Autodesk Fusion 360 part; units mm, degrees
(part 4 of 8)
  spline S174 degree 5 poles (79.544, 19.9185) (79.5234, 19.9219) (79.4821, 19.9288) (79.4202, 19.939) (79.3377, 19.9523) (79.2346, 19.9687) (79.1314, 19.9847) (79.0284, 20.0004) (78.9253, 20.0157) (78.8222, 20.0307) (78.7192, 20.0453) (78.6162, 20.0596) (78.5133, 20.0735) (78.4103, 20.087) (78.3074, 20.1002) (78.2045, 20.113) (78.1017, 20.1254) (77.9989, 20.1375) (77.8961, 20.1491) (77.7934, 20.1604) (77.6906, 20.1714) (77.588, 20.1819) (77.4853, 20.192) (77.3827, 20.2018) (77.2802, 20.2111) (77.1777, 20.2201) (77.0752, 20.2287) (76.9728, 20.2368) (76.8704, 20.2446) (76.768, 20.2519) (76.6658, 20.2588) (76.5635, 20.2653) (76.4613, 20.2714) (76.3592, 20.277) (76.2571, 20.2822) (76.1551, 20.287) (76.0531, 20.2913) (75.9512, 20.2952) (75.8646, 20.2981) (75.7985, 20.3001) (75.7526, 20.3014) (75.7272, 20.302) (75.722, 20.3022) knots -1 -1 -1 -1 -1 -1 -0.985714 -0.971429 -0.957143 -0.942857 -0.928571 -0.914286 -0.9 -0.885714 -0.871429 -0.857143 -0.842857 -0.828571 -0.814286 -0.8 -0.785714 -0.771429 -0.757143 -0.742857 -0.728571 -0.714286 -0.7 -0.685714 -0.671429 -0.657143 -0.642857 -0.628571 -0.614286 -0.6 -0.585714 -0.571429 -0.557143 -0.542857 -0.528571 -0.514286 -0.5 -0.485714 -0.471429 -0.467834 -0.467834 -0.467834 -0.467834 -0.467834 -0.467834
  spline S175 degree 3 poles (74.7851, 21.0311) (74.8203, 20.9058) (74.8797, 20.7885) (75.0401, 20.5833) (75.1396, 20.4974) (75.3241, 20.3923) (75.4002, 20.3606) (75.5584, 20.3165) (75.6399, 20.3043) (75.722, 20.3022) knots 0 0 0 0 0.039064 0.039064 0.078129 0.078129 0.102767 0.102767 0.127404 0.127404 0.127404 0.127404
  arc A88 (74.7851, 21.0311) -> (74.7535, 21.1431) centre (0, 0) ccw
  spline S176 degree 3 poles (75.1715, 22.2542) (75.0623, 22.1834) (74.9679, 22.0918) (74.8196, 21.8778) (74.767, 21.7573) (74.7214, 21.5499) (74.7137, 21.4678) (74.7186, 21.3036) (74.7311, 21.2221) (74.7535, 21.1431) knots 0 0 0 0 0.039064 0.039064 0.078129 0.078129 0.102767 0.102767 0.127404 0.127404 0.127404 0.127404
  spline S177 degree 5 poles (75.1715, 22.2542) (75.1758, 22.257) (75.1972, 22.2709) (75.2356, 22.2959) (75.291, 22.3322) (75.3633, 22.3799) (75.4482, 22.4364) (75.5328, 22.4934) (75.6173, 22.5508) (75.7016, 22.6086) (75.7858, 22.6667) (75.8697, 22.7253) (75.9535, 22.7843) (76.0371, 22.8436) (76.1205, 22.9033) (76.2038, 22.9634) (76.2868, 23.0239) (76.3697, 23.0847) (76.4525, 23.1459) (76.535, 23.2075) (76.6174, 23.2694) (76.6996, 23.3317) (76.7817, 23.3943) (76.8635, 23.4573) (76.9452, 23.5206) (77.0268, 23.5843) (77.1081, 23.6483) (77.1893, 23.7126) (77.2704, 23.7773) (77.3512, 23.8423) (77.4319, 23.9076) (77.5125, 23.9733) (77.5928, 24.0392) (77.673, 24.1055) (77.7531, 24.1721) (77.8329, 24.239) (77.9127, 24.3063) (77.9922, 24.3738) (78.0716, 24.4417) (78.135, 24.4962) (78.1824, 24.5372) (78.214, 24.5646) (78.2298, 24.5784) knots 0.467834 0.467834 0.467834 0.467834 0.467834 0.467834 0.471429 0.485714 0.5 0.514286 0.528571 0.542857 0.557143 0.571429 0.585714 0.6 0.614286 0.628571 0.642857 0.657143 0.671429 0.685714 0.7 0.714286 0.728571 0.742857 0.757143 0.771429 0.785714 0.8 0.814286 0.828571 0.842857 0.857143 0.871429 0.885714 0.9 0.914286 0.928571 0.942857 0.957143 0.971429 0.985714 1 1 1 1 1 1
  arc A89 (78.2298, 24.5784) -> (77.736, 26.098) centre (0, 0) ccw
  spline S178 degree 5 poles (77.736, 26.098) (77.7152, 26.0998) (77.6735, 26.1034) (77.611, 26.1087) (77.5277, 26.1156) (77.4236, 26.1238) (77.3195, 26.1317) (77.2155, 26.1393) (77.1116, 26.1464) (77.0077, 26.1533) (76.9038, 26.1598) (76.8, 26.1659) (76.6963, 26.1717) (76.5926, 26.1771) (76.489, 26.1821) (76.3854, 26.1868) (76.2819, 26.1912) (76.1785, 26.1951) (76.0751, 26.1987) (75.9718, 26.2019) (75.8685, 26.2047) (75.7653, 26.2072) (75.6622, 26.2092) (75.5592, 26.2109) (75.4562, 26.2122) (75.3533, 26.2131) (75.2505, 26.2136) (75.1477, 26.2136) (75.045, 26.2133) (74.9424, 26.2126) (74.8399, 26.2115) (74.7375, 26.2099) (74.6352, 26.208) (74.5329, 26.2056) (74.4307, 26.2028) (74.3286, 26.1995) (74.2267, 26.1959) (74.1248, 26.1917) (74.0382, 26.1878) (73.9721, 26.1846) (73.9263, 26.1823) (73.9008, 26.1809) (73.8957, 26.1807) knots -1 -1 -1 -1 -1 -1 -0.985714 -0.971429 -0.957143 -0.942857 -0.928571 -0.914286 -0.9 -0.885714 -0.871429 -0.857143 -0.842857 -0.828571 -0.814286 -0.8 -0.785714 -0.771429 -0.757143 -0.742857 -0.728571 -0.714286 -0.7 -0.685714 -0.671429 -0.657143 -0.642857 -0.628571 -0.614286 -0.6 -0.585714 -0.571429 -0.557143 -0.542857 -0.528571 -0.514286 -0.5 -0.485714 -0.471429 -0.467834 -0.467834 -0.467834 -0.467834 -0.467834 -0.467834
  spline S179 degree 3 poles (72.9045, 26.8339) (72.9494, 26.7117) (73.0178, 26.5994) (73.1939, 26.4075) (73.2998, 26.3296) (73.4919, 26.2393) (73.5703, 26.2136) (73.7315, 26.1821) (73.8137, 26.1763) (73.8957, 26.1807) knots 0 0 0 0 0.039064 0.039064 0.078129 0.078129 0.102767 0.102767 0.127404 0.127404 0.127404 0.127404
  arc A90 (72.9045, 26.8339) -> (72.8642, 26.943) centre (0, 0) ccw
  spline S180 degree 3 poles (73.1937, 28.0835) (73.0904, 28.0043) (73.0035, 27.9056) (72.8724, 27.6806) (72.8295, 27.5563) (72.8003, 27.346) (72.7991, 27.2636) (72.8168, 27.1003) (72.8357, 27.0201) (72.8642, 26.943) knots 0 0 0 0 0.039064 0.039064 0.078129 0.078129 0.102767 0.102767 0.127404 0.127404 0.127404 0.127404
  spline S181 degree 5 poles (73.1937, 28.0835) (73.1978, 28.0866) (73.218, 28.1021) (73.2543, 28.1301) (73.3067, 28.1706) (73.3751, 28.2238) (73.4552, 28.2869) (73.5352, 28.3503) (73.6149, 28.4141) (73.6944, 28.4784) (73.7737, 28.543) (73.8528, 28.6079) (73.9317, 28.6733) (74.0104, 28.739) (74.0889, 28.8051) (74.1672, 28.8715) (74.2452, 28.9383) (74.3231, 29.0055) (74.4008, 29.073) (74.4783, 29.1408) (74.5555, 29.209) (74.6326, 29.2776) (74.7095, 29.3464) (74.7861, 29.4156) (74.8626, 29.4852) (74.9389, 29.555) (75.015, 29.6252) (75.0909, 29.6957) (75.1666, 29.7666) (75.2421, 29.8377) (75.3175, 29.9091) (75.3926, 29.9809) (75.4675, 30.053) (75.5423, 30.1254) (75.6169, 30.198) (75.6912, 30.271) (75.7654, 30.3443) (75.8394, 30.4179) (75.9132, 30.4917) (75.9721, 30.5511) (76.0162, 30.5957) (76.0456, 30.6255) (76.0603, 30.6404) knots 0.467834 0.467834 0.467834 0.467834 0.467834 0.467834 0.471429 0.485714 0.5 0.514286 0.528571 0.542857 0.557143 0.571429 0.585714 0.6 0.614286 0.628571 0.642857 0.657143 0.671429 0.685714 0.7 0.714286 0.728571 0.742857 0.757143 0.771429 0.785714 0.8 0.814286 0.828571 0.842857 0.857143 0.871429 0.885714 0.9 0.914286 0.928571 0.942857 0.957143 0.971429 0.985714 1 1 1 1 1 1
  arc A91 (76.0603, 30.6404) -> (75.4488, 32.1167) centre (0, 0) ccw
  spline S182 degree 5 poles (75.4488, 32.1167) (75.4279, 32.1168) (75.386, 32.1172) (75.3233, 32.1175) (75.2397, 32.1178) (75.1353, 32.1179) (75.0309, 32.1176) (74.9266, 32.1169) (74.8224, 32.116) (74.7183, 32.1146) (74.6143, 32.1129) (74.5103, 32.1109) (74.4065, 32.1085) (74.3027, 32.1058) (74.199, 32.1027) (74.0953, 32.0992) (73.9918, 32.0954) (73.8884, 32.0912) (73.785, 32.0867) (73.6818, 32.0818) (73.5786, 32.0765) (73.4756, 32.0708) (73.3726, 32.0648) (73.2698, 32.0584) (73.167, 32.0516) (73.0644, 32.0444) (72.9618, 32.0368) (72.8594, 32.0289) (72.757, 32.0205) (72.6548, 32.0117) (72.5527, 32.0026) (72.4507, 31.993) (72.3488, 31.983) (72.2471, 31.9726) (72.1454, 31.9618) (72.0439, 31.9505) (71.9425, 31.9389) (71.8413, 31.9267) (71.7553, 31.9161) (71.6896, 31.9077) (71.6442, 31.9018) (71.6189, 31.8984) (71.6138, 31.8977) knots -1 -1 -1 -1 -1 -1 -0.985714 -0.971429 -0.957143 -0.942857 -0.928571 -0.914286 -0.9 -0.885714 -0.871429 -0.857143 -0.842857 -0.828571 -0.814286 -0.8 -0.785714 -0.771429 -0.757143 -0.742857 -0.728571 -0.714286 -0.7 -0.685714 -0.671429 -0.657143 -0.642857 -0.628571 -0.614286 -0.6 -0.585714 -0.571429 -0.557143 -0.542857 -0.528571 -0.514286 -0.5 -0.485714 -0.471429 -0.467834 -0.467834 -0.467834 -0.467834 -0.467834 -0.467834
  spline S183 degree 3 poles (70.5744, 32.4711) (70.6288, 32.3529) (70.7058, 32.2463) (70.8963, 32.0688) (71.008, 31.9995) (71.2067, 31.9245) (71.2868, 31.9051) (71.45, 31.8863) (71.5324, 31.887) (71.6138, 31.8977) knots 0 0 0 0 0.039064 0.039064 0.078129 0.078129 0.102767 0.102767 0.127404 0.127404 0.127404 0.127404
  arc A92 (70.5744, 32.4711) -> (70.5256, 32.5768) centre (0, 0) ccw
  spline S184 degree 3 poles (70.7647, 33.7396) (70.6679, 33.6526) (70.589, 33.5474) (70.476, 33.3128) (70.443, 33.1855) (70.4303, 32.9736) (70.4356, 32.8913) (70.4661, 32.7299) (70.4912, 32.6514) (70.5256, 32.5768) knots 0 0 0 0 0.039064 0.039064 0.078129 0.078129 0.102767 0.102767 0.127404 0.127404 0.127404 0.127404
  spline S185 degree 5 poles (70.7647, 33.7396) (70.7685, 33.7431) (70.7874, 33.7601) (70.8215, 33.7908) (70.8705, 33.8353) (70.9345, 33.8938) (71.0094, 33.9629) (71.0842, 34.0324) (71.1586, 34.1023) (71.2329, 34.1726) (71.3069, 34.2432) (71.3806, 34.3142) (71.4541, 34.3855) (71.5274, 34.4572) (71.6005, 34.5292) (71.6733, 34.6016) (71.7459, 34.6743) (71.8183, 34.7474) (71.8904, 34.8208) (71.9623, 34.8945) (72.034, 34.9686) (72.1054, 35.0429) (72.1767, 35.1176) (72.2477, 35.1926) (72.3185, 35.2679) (72.389, 35.3436) (72.4594, 35.4195) (72.5295, 35.4958) (72.5995, 35.5723) (72.6692, 35.6491) (72.7386, 35.7263) (72.8079, 35.8037) (72.877, 35.8815) (72.9458, 35.9595) (73.0144, 36.0378) (73.0829, 36.1164) (73.1511, 36.1952) (73.2191, 36.2744) (73.2869, 36.3538) (73.3409, 36.4176) (73.3814, 36.4656) (73.4083, 36.4976) (73.4218, 36.5136) knots 0.467834 0.467834 0.467834 0.467834 0.467834 0.467834 0.471429 0.485714 0.5 0.514286 0.528571 0.542857 0.557143 0.571429 0.585714 0.6 0.614286 0.628571 0.642857 0.657143 0.671429 0.685714 0.7 0.714286 0.728571 0.742857 0.757143 0.771429 0.785714 0.8 0.814286 0.828571 0.842857 0.857143 0.871429 0.885714 0.9 0.914286 0.928571 0.942857 0.957143 0.971429 0.985714 1 1 1 1 1 1
  arc A93 (73.4218, 36.5136) -> (72.6964, 37.9373) centre (0, 0) ccw
  spline S186 degree 5 poles (72.6964, 37.9373) (72.6755, 37.9358) (72.6338, 37.9329) (72.5712, 37.9283) (72.4878, 37.9221) (72.3837, 37.9139) (72.2797, 37.9054) (72.1758, 37.8966) (72.072, 37.8875) (71.9683, 37.878) (71.8647, 37.8681) (71.7612, 37.8579) (71.6579, 37.8474) (71.5546, 37.8365) (71.4515, 37.8253) (71.3485, 37.8137) (71.2456, 37.8018) (71.1428, 37.7895) (71.0401, 37.7769) (70.9376, 37.7639) (70.8351, 37.7505) (70.7328, 37.7368) (70.6307, 37.7227) (70.5286, 37.7082) (70.4267, 37.6934) (70.3249, 37.6782) (70.2233, 37.6626) (70.1218, 37.6466) (70.0204, 37.6302) (69.9192, 37.6135) (69.8182, 37.5963) (69.7172, 37.5788) (69.6164, 37.5608) (69.5158, 37.5425) (69.4153, 37.5237) (69.315, 37.5045) (69.2149, 37.4849) (69.1149, 37.4649) (69.03, 37.4475) (68.9652, 37.434) (68.9203, 37.4245) (68.8954, 37.4192) (68.8904, 37.4182) knots -1 -1 -1 -1 -1 -1 -0.985714 -0.971429 -0.957143 -0.942857 -0.928571 -0.914286 -0.9 -0.885714 -0.871429 -0.857143 -0.842857 -0.828571 -0.814286 -0.8 -0.785714 -0.771429 -0.757143 -0.742857 -0.728571 -0.714286 -0.7 -0.685714 -0.671429 -0.657143 -0.642857 -0.628571 -0.614286 -0.6 -0.585714 -0.571429 -0.557143 -0.542857 -0.528571 -0.514286 -0.5 -0.485714 -0.471429 -0.467834 -0.467834 -0.467834 -0.467834 -0.467834 -0.467834
  spline S187 degree 3 poles (67.8091, 37.9083) (67.8727, 37.7946) (67.9578, 37.6944) (68.1617, 37.5324) (68.2785, 37.472) (68.4824, 37.4129) (68.5638, 37.3998) (68.7279, 37.3939) (68.8101, 37.4011) (68.8904, 37.4182) knots 0 0 0 0 0.039064 0.039064 0.078129 0.078129 0.102767 0.102767 0.127404 0.127404 0.127404 0.127404
  arc A94 (67.8091, 37.9083) -> (67.7523, 38.0098) centre (0, 0) ccw
  spline S188 degree 3 poles (67.8994, 39.1878) (67.8097, 39.0934) (67.7393, 38.9823) (67.6451, 38.7396) (67.6221, 38.6101) (67.6262, 38.3978) (67.6378, 38.3162) (67.6809, 38.1577) (67.7121, 38.0814) (67.7523, 38.0098) knots 0 0 0 0 0.039064 0.039064 0.078129 0.078129 0.102767 0.102767 0.127404 0.127404 0.127404 0.127404
  spline S189 degree 5 poles (67.8994, 39.1878) (67.9029, 39.1915) (67.9204, 39.21) (67.9519, 39.2433) (67.9974, 39.2915) (68.0565, 39.3548) (68.1258, 39.4296) (68.1949, 39.5047) (68.2636, 39.5802) (68.3321, 39.6561) (68.4004, 39.7323) (68.4683, 39.8088) (68.536, 39.8857) (68.6035, 39.963) (68.6706, 40.0405) (68.7376, 40.1184) (68.8042, 40.1966) (68.8706, 40.2751) (68.9368, 40.3539) (69.0027, 40.433) (69.0683, 40.5125) (69.1337, 40.5922) (69.1989, 40.6723) (69.2638, 40.7526) (69.3285, 40.8333) (69.3929, 40.9142) (69.457, 40.9954) (69.521, 41.0769) (69.5847, 41.1587) (69.6481, 41.2408) (69.7114, 41.3232) (69.7743, 41.4058) (69.8371, 41.4887) (69.8996, 41.5719) (69.9619, 41.6553) (70.0239, 41.7391) (70.0857, 41.823) (70.1473, 41.9073) (70.2087, 41.9918) (70.2576, 42.0596) (70.2941, 42.1106) (70.3185, 42.1446) (70.3306, 42.1616) knots 0.467834 0.467834 0.467834 0.467834 0.467834 0.467834 0.471429 0.485714 0.5 0.514286 0.528571 0.542857 0.557143 0.571429 0.585714 0.6 0.614286 0.628571 0.642857 0.657143 0.671429 0.685714 0.7 0.714286 0.728571 0.742857 0.757143 0.771429 0.785714 0.8 0.814286 0.828571 0.842857 0.857143 0.871429 0.885714 0.9 0.914286 0.928571 0.942857 0.957143 0.971429 0.985714 1 1 1 1 1 1
  arc A95 (70.3306, 42.1616) -> (69.4957, 43.524) centre (0, 0) ccw
  spline S190 degree 5 poles (69.4957, 43.524) (69.475, 43.521) (69.4337, 43.5147) (69.3716, 43.5053) (69.289, 43.4925) (69.1859, 43.4762) (69.0829, 43.4596) (68.98, 43.4426) (68.8772, 43.4254) (68.7746, 43.4078) (68.6721, 43.3898) (68.5697, 43.3716) (68.4675, 43.353) (68.3654, 43.334) (68.2635, 43.3147) (68.1617, 43.2951) (68.06, 43.2752) (67.9585, 43.2548) (67.8572, 43.2342) (67.756, 43.2132) (67.6549, 43.1918) (67.554, 43.1701) (67.4532, 43.148) (67.3527, 43.1256) (67.2522, 43.1028) (67.152, 43.0797) (67.0519, 43.0561) (66.9519, 43.0322) (66.8522, 43.008) (66.7526, 42.9833) (66.6532, 42.9583) (66.5539, 42.9329) (66.4549, 42.9071) (66.356, 42.8809) (66.2573, 42.8543) (66.1588, 42.8273) (66.0605, 42.7999) (65.9624, 42.7721) (65.8791, 42.7481) (65.8155, 42.7296) (65.7716, 42.7166) (65.7471, 42.7094) (65.7422, 42.7079) knots -1 -1 -1 -1 -1 -1 -0.985714 -0.971429 -0.957143 -0.942857 -0.928571 -0.914286 -0.9 -0.885714 -0.871429 -0.857143 -0.842857 -0.828571 -0.814286 -0.8 -0.785714 -0.771429 -0.757143 -0.742857 -0.728571 -0.714286 -0.7 -0.685714 -0.671429 -0.657143 -0.642857 -0.628571 -0.614286 -0.6 -0.585714 -0.571429 -0.557143 -0.542857 -0.528571 -0.514286 -0.5 -0.485714 -0.471429 -0.467834 -0.467834 -0.467834 -0.467834 -0.467834 -0.467834
  spline S191 degree 3 poles (64.6259, 43.1116) (64.6981, 43.0033) (64.7908, 42.9101) (65.0068, 42.7646) (65.128, 42.7136) (65.3359, 42.6706) (65.4181, 42.664) (65.5822, 42.671) (65.6635, 42.6845) (65.7422, 42.7079) knots 0 0 0 0 0.039064 0.039064 0.078129 0.078129 0.102767 0.102767 0.127404 0.127404 0.127404 0.127404
  arc A96 (64.6259, 43.1116) -> (64.5612, 43.2084) centre (0, 0) ccw
  spline S192 degree 3 poles (64.6154, 44.3943) (64.5334, 44.2931) (64.472, 44.1769) (64.3971, 43.9275) (64.3843, 43.7967) (64.405, 43.5853) (64.4231, 43.5049) (64.4784, 43.3503) (64.5155, 43.2766) (64.5612, 43.2084) knots 0 0 0 0 0.039064 0.039064 0.078129 0.078129 0.102767 0.102767 0.127404 0.127404 0.127404 0.127404
  spline S193 degree 5 poles (64.6154, 44.3943) (64.6186, 44.3983) (64.6347, 44.4181) (64.6635, 44.4537) (64.705, 44.5053) (64.759, 44.5731) (64.8222, 44.6531) (64.8852, 44.7334) (64.9478, 44.8141) (65.0101, 44.8951) (65.0721, 44.9764) (65.1339, 45.0581) (65.1954, 45.1401) (65.2565, 45.2223) (65.3174, 45.3049) (65.378, 45.3878) (65.4383, 45.471) (65.4984, 45.5544) (65.5581, 45.6382) (65.6176, 45.7223) (65.6768, 45.8066) (65.7358, 45.8913) (65.7945, 45.9762) (65.8529, 46.0614) (65.911, 46.1468) (65.9689, 46.2326) (66.0265, 46.3186) (66.0838, 46.4049) (66.1409, 46.4914) (66.1977, 46.5782) (66.2543, 46.6653) (66.3106, 46.7526) (66.3666, 46.8402) (66.4224, 46.928) (66.478, 47.0161) (66.5333, 47.1044) (66.5883, 47.193) (66.6431, 47.2818) (66.6976, 47.3708) (66.741, 47.4423) (66.7735, 47.496) (66.7951, 47.5318) (66.8058, 47.5498) knots 0.467834 0.467834 0.467834 0.467834 0.467834 0.467834 0.471429 0.485714 0.5 0.514286 0.528571 0.542857 0.557143 0.571429 0.585714 0.6 0.614286 0.628571 0.642857 0.657143 0.671429 0.685714 0.7 0.714286 0.728571 0.742857 0.757143 0.771429 0.785714 0.8 0.814286 0.828571 0.842857 0.857143 0.871429 0.885714 0.9 0.914286 0.928571 0.942857 0.957143 0.971429 0.985714 1 1 1 1 1 1
  arc A97 (66.8058, 47.5498) -> (65.8666, 48.8425) centre (0, 0) ccw
  spline S194 degree 5 poles (65.8666, 48.8425) (65.8463, 48.8377) (65.8055, 48.8283) (65.7444, 48.814) (65.663, 48.7948) (65.5615, 48.7704) (65.4601, 48.7458) (65.3589, 48.7208) (65.2578, 48.6955) (65.1568, 48.6699) (65.0561, 48.644) (64.9555, 48.6178) (64.855, 48.5912) (64.7547, 48.5643) (64.6546, 48.5371) (64.5547, 48.5096) (64.4549, 48.4817) (64.3553, 48.4535) (64.2559, 48.4249) (64.1566, 48.396) (64.0575, 48.3668) (63.9587, 48.3373) (63.86, 48.3074) (63.7614, 48.2771) (63.6631, 48.2465) (63.565, 48.2156) (63.467, 48.1842) (63.3693, 48.1526) (63.2717, 48.1206) (63.1744, 48.0882) (63.0772, 48.0554) (62.9803, 48.0223) (62.8835, 47.9888) (62.787, 47.9549) (62.6907, 47.9207) (62.5946, 47.8861) (62.4988, 47.851) (62.4032, 47.8156) (62.322, 47.7852) (62.2601, 47.7617) (62.2173, 47.7453) (62.1935, 47.7362) (62.1887, 47.7343) knots -1 -1 -1 -1 -1 -1 -0.985714 -0.971429 -0.957143 -0.942857 -0.928571 -0.914286 -0.9 -0.885714 -0.871429 -0.857143 -0.842857 -0.828571 -0.814286 -0.8 -0.785714 -0.771429 -0.757143 -0.742857 -0.728571 -0.714286 -0.7 -0.685714 -0.671429 -0.657143 -0.642857 -0.628571 -0.614286 -0.6 -0.585714 -0.571429 -0.557143 -0.542857 -0.528571 -0.514286 -0.5 -0.485714 -0.471429 -0.467834 -0.467834 -0.467834 -0.467834 -0.467834 -0.467834
  spline S195 degree 3 poles (61.0441, 48.0492) (61.1247, 47.9469) (61.2244, 47.8613) (61.4511, 47.7331) (61.5759, 47.6918) (61.7866, 47.6653) (61.869, 47.6651) (62.0321, 47.6849) (62.1121, 47.7049) (62.1887, 47.7343) knots 0 0 0 0 0.039064 0.039064 0.078129 0.078129 0.102767 0.102767 0.127404 0.127404 0.127404 0.127404
  arc A98 (61.0441, 48.0492) -> (60.9721, 48.1406) centre (0, 0) ccw
  spline S196 degree 3 poles (60.9331, 49.3271) (60.8593, 49.2198) (60.8071, 49.0992) (60.752, 48.8446) (60.7496, 48.7132) (60.7868, 48.5041) (60.8111, 48.4254) (60.8784, 48.2756) (60.9212, 48.2051) (60.9721, 48.1406) knots 0 0 0 0 0.039064 0.039064 0.078129 0.078129 0.102767 0.102767 0.127404 0.127404 0.127404 0.127404
  spline S197 degree 5 poles (60.9331, 49.3271) (60.936, 49.3313) (60.9504, 49.3523) (60.9764, 49.3901) (61.0137, 49.4448) (61.0622, 49.5166) (61.119, 49.6013) (61.1754, 49.6864) (61.2315, 49.7717) (61.2873, 49.8574) (61.3427, 49.9433) (61.3979, 50.0295) (61.4527, 50.1161) (61.5073, 50.2029) (61.5615, 50.29) (61.6154, 50.3774) (61.669, 50.465) (61.7223, 50.553) (61.7753, 50.6412) (61.828, 50.7296) (61.8804, 50.8184) (61.9325, 50.9074) (61.9844, 50.9966) (62.0359, 51.0861) (62.0872, 51.1759) (62.1381, 51.2659) (62.1888, 51.3562) (62.2392, 51.4467) (62.2893, 51.5374) (62.3392, 51.6284) (62.3887, 51.7197) (62.438, 51.8111) (62.487, 51.9028) (62.5357, 51.9948) (62.5842, 52.0869) (62.6324, 52.1793) (62.6803, 52.2719) (62.7279, 52.3648) (62.7753, 52.4579) (62.813, 52.5325) (62.8411, 52.5886) (62.8599, 52.626) (62.8692, 52.6447) knots 0.467834 0.467834 0.467834 0.467834 0.467834 0.467834 0.471429 0.485714 0.5 0.514286 0.528571 0.542857 0.557143 0.571429 0.585714 0.6 0.614286 0.628571 0.642857 0.657143 0.671429 0.685714 0.7 0.714286 0.728571 0.742857 0.757143 0.771429 0.785714 0.8 0.814286 0.828571 0.842857 0.857143 0.871429 0.885714 0.9 0.914286 0.928571 0.942857 0.957143 0.971429 0.985714 1 1 1 1 1 1
  arc A99 (62.8692, 52.6447) -> (61.8315, 53.8597) centre (0, 0) ccw
  spline S198 degree 5 poles (61.8315, 53.8597) (61.8115, 53.8534) (61.7716, 53.8408) (61.7118, 53.8218) (61.6322, 53.7962) (61.5329, 53.764) (61.4338, 53.7315) (61.3348, 53.6986) (61.236, 53.6655) (61.1374, 53.632) (61.039, 53.5983) (60.9407, 53.5642) (60.8427, 53.5299) (60.7448, 53.4952) (60.6471, 53.4602) (60.5497, 53.4249) (60.4524, 53.3893) (60.3553, 53.3534) (60.2584, 53.3171) (60.1617, 53.2805) (60.0653, 53.2436) (59.969, 53.2064) (59.8729, 53.1688) (59.7771, 53.1309) (59.6815, 53.0927) (59.5861, 53.0542) (59.4909, 53.0153) (59.3959, 52.976) (59.3012, 52.9365) (59.2067, 52.8965) (59.1124, 52.8563) (59.0183, 52.8156) (58.9245, 52.7747) (58.831, 52.7333) (58.7377, 52.6916) (58.6446, 52.6496) (58.5518, 52.6071) (58.4592, 52.5643) (58.3807, 52.5276) (58.3209, 52.4993) (58.2795, 52.4796) (58.2565, 52.4687) (58.2518, 52.4665) knots -1 -1 -1 -1 -1 -1 -0.985714 -0.971429 -0.957143 -0.942857 -0.928571 -0.914286 -0.9 -0.885714 -0.871429 -0.857143 -0.842857 -0.828571 -0.814286 -0.8 -0.785714 -0.771429 -0.757143 -0.742857 -0.728571 -0.714286 -0.7 -0.685714 -0.671429 -0.657143 -0.642857 -0.628571 -0.614286 -0.6 -0.585714 -0.571429 -0.557143 -0.542857 -0.528571 -0.514286 -0.5 -0.485714 -0.471429 -0.467834 -0.467834 -0.467834 -0.467834 -0.467834 -0.467834
  spline S199 degree 3 poles (57.0861, 52.6906) (57.1744, 52.5949) (57.2805, 52.5174) (57.5166, 52.4074) (57.6443, 52.376) (57.8564, 52.3661) (57.9386, 52.3724) (58.0996, 52.4049) (58.1777, 52.4311) (58.2518, 52.4665) knots 0 0 0 0 0.039064 0.039064 0.078129 0.078129 0.102767 0.102767 0.127404 0.127404 0.127404 0.127404
  arc A100 (57.0861, 52.6906) -> (57.0071, 52.776) centre (0, 0) ccw
  spline S200 degree 3 poles (56.8751, 53.9558) (56.8099, 53.8431) (56.7674, 53.7187) (56.7325, 53.4606) (56.7403, 53.3294) (56.7938, 53.1239) (56.8243, 53.0473) (56.9031, 52.9032) (56.9513, 52.8363) (57.0071, 52.776) knots 0 0 0 0 0.039064 0.039064 0.078129 0.078129 0.102767 0.102767 0.127404 0.127404 0.127404 0.127404
  spline S201 degree 5 poles (56.8751, 53.9558) (56.8777, 53.9602) (56.8904, 53.9823) (56.9133, 54.022) (56.9462, 54.0795) (56.9889, 54.1549) (57.0389, 54.2438) (57.0885, 54.333) (57.1377, 54.4224) (57.1866, 54.5122) (57.2351, 54.6022) (57.2834, 54.6925) (57.3312, 54.7831) (57.3788, 54.8739) (57.426, 54.965) (57.4729, 55.0564) (57.5194, 55.148) (57.5657, 55.2398) (57.6116, 55.3319) (57.6572, 55.4242) (57.7025, 55.5168) (57.7475, 55.6096) (57.7922, 55.7027) (57.8365, 55.7959) (57.8806, 55.8894) (57.9243, 55.9832) (57.9678, 56.0771) (58.0109, 56.1713) (58.0537, 56.2657) (58.0963, 56.3604) (58.1385, 56.4552) (58.1805, 56.5503) (58.2221, 56.6455) (58.2635, 56.741) (58.3046, 56.8367) (58.3454, 56.9326) (58.3859, 57.0287) (58.4261, 57.1249) (58.466, 57.2214) (58.4977, 57.2988) (58.5214, 57.3569) (58.5371, 57.3957) (58.5449, 57.4151) knots 0.467834 0.467834 0.467834 0.467834 0.467834 0.467834 0.471429 0.485714 0.5 0.514286 0.528571 0.542857 0.557143 0.571429 0.585714 0.6 0.614286 0.628571 0.642857 0.657143 0.671429 0.685714 0.7 0.714286 0.728571 0.742857 0.757143 0.771429 0.785714 0.8 0.814286 0.828571 0.842857 0.857143 0.871429 0.885714 0.9 0.914286 0.928571 0.942857 0.957143 0.971429 0.985714 1 1 1 1 1 1
  arc A101 (58.5449, 57.4151) -> (57.4151, 58.5449) centre (0, 0) ccw
  spline S202 degree 5 poles (57.4151, 58.5449) (57.3957, 58.5371) (57.3569, 58.5214) (57.2988, 58.4977) (57.2214, 58.466) (57.1249, 58.4261) (57.0287, 58.3859) (56.9326, 58.3454) (56.8367, 58.3046) (56.741, 58.2635) (56.6455, 58.2221) (56.5503, 58.1805) (56.4552, 58.1385) (56.3604, 58.0963) (56.2657, 58.0537) (56.1713, 58.0109) (56.0771, 57.9678) (55.9832, 57.9243) (55.8894, 57.8806) (55.7959, 57.8365) (55.7027, 57.7922) (55.6096, 57.7475) (55.5168, 57.7025) (55.4242, 57.6572) (55.3319, 57.6116) (55.2398, 57.5657) (55.148, 57.5194) (55.0564, 57.4729) (54.965, 57.426) (54.8739, 57.3788) (54.7831, 57.3312) (54.6925, 57.2834) (54.6022, 57.2351) (54.5122, 57.1866) (54.4224, 57.1377) (54.333, 57.0885) (54.2438, 57.0389) (54.1549, 56.9889) (54.0795, 56.9462) (54.022, 56.9133) (53.9823, 56.8904) (53.9602, 56.8777) (53.9558, 56.8751) knots -1 -1 -1 -1 -1 -1 -0.985714 -0.971429 -0.957143 -0.942857 -0.928571 -0.914286 -0.9 -0.885714 -0.871429 -0.857143 -0.842857 -0.828571 -0.814286 -0.8 -0.785714 -0.771429 -0.757143 -0.742857 -0.728571 -0.714286 -0.7 -0.685714 -0.671429 -0.657143 -0.642857 -0.628571 -0.614286 -0.6 -0.585714 -0.571429 -0.557143 -0.542857 -0.528571 -0.514286 -0.5 -0.485714 -0.471429 -0.467834 -0.467834 -0.467834 -0.467834 -0.467834 -0.467834
  spline S203 degree 3 poles (52.776, 57.0071) (52.8716, 56.9186) (52.9835, 56.8497) (53.2275, 56.7585) (53.3572, 56.7372) (53.5694, 56.744) (53.6509, 56.7567) (53.8088, 56.8018) (53.8847, 56.834) (53.9558, 56.8751) knots 0 0 0 0 0.039064 0.039064 0.078129 0.078129 0.102767 0.102767 0.127404 0.127404 0.127404 0.127404
  arc A102 (52.776, 57.0071) -> (52.6906, 57.0861) centre (0, 0) ccw
  spline S204 degree 3 poles (52.4665, 58.2518) (52.4103, 58.1343) (52.3777, 58.007) (52.3631, 57.747) (52.3812, 57.6168) (52.4507, 57.4161) (52.487, 57.3421) (52.577, 57.2047) (52.6302, 57.1418) (52.6906, 57.0861) knots 0 0 0 0 0.039064 0.039064 0.078129 0.078129 0.102767 0.102767 0.127404 0.127404 0.127404 0.127404
  spline S205 degree 5 poles (52.4665, 58.2518) (52.4687, 58.2565) (52.4796, 58.2795) (52.4993, 58.3209) (52.5276, 58.3807) (52.5643, 58.4592) (52.6071, 58.5518) (52.6496, 58.6446) (52.6916, 58.7377) (52.7333, 58.831) (52.7747, 58.9245) (52.8156, 59.0183) (52.8563, 59.1124) (52.8965, 59.2067) (52.9365, 59.3012) (52.976, 59.3959) (53.0153, 59.4909) (53.0542, 59.5861) (53.0927, 59.6815) (53.1309, 59.7771) (53.1688, 59.8729) (53.2064, 59.969) (53.2436, 60.0653) (53.2805, 60.1617) (53.3171, 60.2584) (53.3534, 60.3553) (53.3893, 60.4524) (53.4249, 60.5497) (53.4602, 60.6471) (53.4952, 60.7448) (53.5299, 60.8427) (53.5642, 60.9407) (53.5983, 61.039) (53.632, 61.1374) (53.6655, 61.236) (53.6986, 61.3348) (53.7315, 61.4338) (53.764, 61.5329) (53.7962, 61.6322) (53.8218, 61.7118) (53.8408, 61.7716) (53.8534, 61.8115) (53.8597, 61.8315) knots 0.467834 0.467834 0.467834 0.467834 0.467834 0.467834 0.471429 0.485714 0.5 0.514286 0.528571 0.542857 0.557143 0.571429 0.585714 0.6 0.614286 0.628571 0.642857 0.657143 0.671429 0.685714 0.7 0.714286 0.728571 0.742857 0.757143 0.771429 0.785714 0.8 0.814286 0.828571 0.842857 0.857143 0.871429 0.885714 0.9 0.914286 0.928571 0.942857 0.957143 0.971429 0.985714 1 1 1 1 1 1
  arc A103 (53.8597, 61.8315) -> (52.6447, 62.8692) centre (0, 0) ccw
  spline S206 degree 5 poles (52.6447, 62.8692) (52.626, 62.8599) (52.5886, 62.8411) (52.5325, 62.813) (52.4579, 62.7753) (52.3648, 62.7279) (52.2719, 62.6803) (52.1793, 62.6324) (52.0869, 62.5842) (51.9948, 62.5357) (51.9028, 62.487) (51.8111, 62.438) (51.7197, 62.3887) (51.6284, 62.3392) (51.5374, 62.2893) (51.4467, 62.2392) (51.3562, 62.1888) (51.2659, 62.1381) (51.1759, 62.0872) (51.0861, 62.0359) (50.9966, 61.9844) (50.9074, 61.9325) (50.8184, 61.8804) (50.7296, 61.828) (50.6412, 61.7753) (50.553, 61.7223) (50.465, 61.669) (50.3774, 61.6154) (50.29, 61.5615) (50.2029, 61.5073) (50.1161, 61.4527) (50.0295, 61.3979) (49.9433, 61.3427) (49.8574, 61.2873) (49.7717, 61.2315) (49.6864, 61.1754) (49.6013, 61.119) (49.5166, 61.0622) (49.4448, 61.0137) (49.3901, 60.9764) (49.3523, 60.9504) (49.3313, 60.936) (49.3271, 60.9331) knots -1 -1 -1 -1 -1 -1 -0.985714 -0.971429 -0.957143 -0.942857 -0.928571 -0.914286 -0.9 -0.885714 -0.871429 -0.857143 -0.842857 -0.828571 -0.814286 -0.8 -0.785714 -0.771429 -0.757143 -0.742857 -0.728571 -0.714286 -0.7 -0.685714 -0.671429 -0.657143 -0.642857 -0.628571 -0.614286 -0.6 -0.585714 -0.571429 -0.557143 -0.542857 -0.528571 -0.514286 -0.5 -0.485714 -0.471429 -0.467834 -0.467834 -0.467834 -0.467834 -0.467834 -0.467834
  spline S207 degree 3 poles (48.1406, 60.9721) (48.2428, 60.8914) (48.3598, 60.8314) (48.6102, 60.7597) (48.7411, 60.7487) (48.9522, 60.7721) (49.0324, 60.7912) (49.1863, 60.8485) (49.2595, 60.8865) (49.3271, 60.9331) knots 0 0 0 0 0.039064 0.039064 0.078129 0.078129 0.102767 0.102767 0.127404 0.127404 0.127404 0.127404
  arc A104 (48.1406, 60.9721) -> (48.0492, 61.0441) centre (0, 0) ccw
  spline S208 degree 3 poles (47.7343, 62.1887) (47.6876, 62.0672) (47.6651, 61.9377) (47.6709, 61.6773) (47.6992, 61.549) (47.7842, 61.3544) (47.8262, 61.2835) (47.9267, 61.1535) (47.9847, 61.0949) (48.0492, 61.0441) knots 0 0 0 0 0.039064 0.039064 0.078129 0.078129 0.102767 0.102767 0.127404 0.127404 0.127404 0.127404
  spline S209 degree 5 poles (47.7343, 62.1887) (47.7362, 62.1935) (47.7453, 62.2173) (47.7617, 62.2601) (47.7852, 62.322) (47.8156, 62.4032) (47.851, 62.4988) (47.8861, 62.5946) (47.9207, 62.6907) (47.9549, 62.787) (47.9888, 62.8835) (48.0223, 62.9803) (48.0554, 63.0772) (48.0882, 63.1744) (48.1206, 63.2717) (48.1526, 63.3693) (48.1842, 63.467) (48.2156, 63.565) (48.2465, 63.6631) (48.2771, 63.7614) (48.3074, 63.86) (48.3373, 63.9587) (48.3668, 64.0575) (48.396, 64.1566) (48.4249, 64.2559) (48.4535, 64.3553) (48.4817, 64.4549) (48.5096, 64.5547) (48.5371, 64.6546) (48.5643, 64.7547) (48.5912, 64.855) (48.6178, 64.9555) (48.644, 65.0561) (48.6699, 65.1568) (48.6955, 65.2578) (48.7208, 65.3589) (48.7458, 65.4601) (48.7704, 65.5615) (48.7948, 65.663) (48.814, 65.7444) (48.8283, 65.8055) (48.8377, 65.8463) (48.8425, 65.8666) knots 0.467834 0.467834 0.467834 0.467834 0.467834 0.467834 0.471429 0.485714 0.5 0.514286 0.528571 0.542857 0.557143 0.571429 0.585714 0.6 0.614286 0.628571 0.642857 0.657143 0.671429 0.685714 0.7 0.714286 0.728571 0.742857 0.757143 0.771429 0.785714 0.8 0.814286 0.828571 0.842857 0.857143 0.871429 0.885714 0.9 0.914286 0.928571 0.942857 0.957143 0.971429 0.985714 1 1 1 1 1 1
  arc A105 (48.8425, 65.8666) -> (47.5498, 66.8058) centre (0, 0) ccw
  spline S210 degree 5 poles (47.5498, 66.8058) (47.5318, 66.7951) (47.496, 66.7735) (47.4423, 66.741) (47.3708, 66.6976) (47.2818, 66.6431) (47.193, 66.5883) (47.1044, 66.5333) (47.0161, 66.478) (46.928, 66.4224) (46.8402, 66.3666) (46.7526, 66.3106) (46.6653, 66.2543) (46.5782, 66.1977) (46.4914, 66.1409) (46.4049, 66.0838) (46.3186, 66.0265) (46.2326, 65.9689) (46.1468, 65.911) (46.0614, 65.8529) (45.9762, 65.7945) (45.8913, 65.7358) (45.8066, 65.6768) (45.7223, 65.6176) (45.6382, 65.5581) (45.5544, 65.4984) (45.471, 65.4383) (45.3878, 65.378) (45.3049, 65.3174) (45.2223, 65.2565) (45.1401, 65.1954) (45.0581, 65.1339) (44.9764, 65.0721) (44.8951, 65.0101) (44.8141, 64.9478) (44.7334, 64.8852) (44.6531, 64.8222) (44.5731, 64.759) (44.5053, 64.705) (44.4537, 64.6635) (44.4181, 64.6347) (44.3983, 64.6186) (44.3943, 64.6154) knots -1 -1 -1 -1 -1 -1 -0.985714 -0.971429 -0.957143 -0.942857 -0.928571 -0.914286 -0.9 -0.885714 -0.871429 -0.857143 -0.842857 -0.828571 -0.814286 -0.8 -0.785714 -0.771429 -0.757143 -0.742857 -0.728571 -0.714286 -0.7 -0.685714 -0.671429 -0.657143 -0.642857 -0.628571 -0.614286 -0.6 -0.585714 -0.571429 -0.557143 -0.542857 -0.528571 -0.514286 -0.5 -0.485714 -0.471429 -0.467834 -0.467834 -0.467834 -0.467834 -0.467834 -0.467834
  spline S211 degree 3 poles (43.2084, 64.5612) (43.3166, 64.4888) (43.4379, 64.4382) (43.6932, 64.3863) (43.8246, 64.3856) (44.0332, 64.4255) (44.1116, 64.4508) (44.2606, 64.52) (44.3305, 64.5637) (44.3943, 64.6154) knots 0 0 0 0 0.039064 0.039064 0.078129 0.078129 0.102767 0.102767 0.127404 0.127404 0.127404 0.127404
  arc A106 (43.2084, 64.5612) -> (43.1116, 64.6259) centre (0, 0) ccw
  spline S212 degree 3 poles (42.7079, 65.7422) (42.6709, 65.6174) (42.6586, 65.4865) (42.6848, 65.2274) (42.7231, 65.1017) (42.8231, 64.9143) (42.8706, 64.8469) (42.9809, 64.7253) (43.0433, 64.6714) (43.1116, 64.6259) knots 0 0 0 0 0.039064 0.039064 0.078129 0.078129 0.102767 0.102767 0.127404 0.127404 0.127404 0.127404
  spline S213 degree 5 poles (42.7079, 65.7422) (42.7094, 65.7471) (42.7166, 65.7716) (42.7296, 65.8155) (42.7481, 65.8791) (42.7721, 65.9624) (42.7999, 66.0605) (42.8273, 66.1588) (42.8543, 66.2573) (42.8809, 66.356) (42.9071, 66.4549) (42.9329, 66.5539) (42.9583, 66.6532) (42.9833, 66.7526) (43.008, 66.8522) (43.0322, 66.9519) (43.0561, 67.0519) (43.0797, 67.152) (43.1028, 67.2522) (43.1256, 67.3527) (43.148, 67.4532) (43.1701, 67.554) (43.1918, 67.6549) (43.2132, 67.756) (43.2342, 67.8572) (43.2548, 67.9585) (43.2752, 68.06) (43.2951, 68.1617) (43.3147, 68.2635) (43.334, 68.3654) (43.353, 68.4675) (43.3716, 68.5697) (43.3898, 68.6721) (43.4078, 68.7746) (43.4254, 68.8772) (43.4426, 68.98) (43.4596, 69.0829) (43.4762, 69.1859) (43.4925, 69.289) (43.5053, 69.3716) (43.5147, 69.4337) (43.521, 69.475) (43.524, 69.4957) knots 0.467834 0.467834 0.467834 0.467834 0.467834 0.467834 0.471429 0.485714 0.5 0.514286 0.528571 0.542857 0.557143 0.571429 0.585714 0.6 0.614286 0.628571 0.642857 0.657143 0.671429 0.685714 0.7 0.714286 0.728571 0.742857 0.757143 0.771429 0.785714 0.8 0.814286 0.828571 0.842857 0.857143 0.871429 0.885714 0.9 0.914286 0.928571 0.942857 0.957143 0.971429 0.985714 1 1 1 1 1 1
  arc A107 (43.524, 69.4957) -> (42.1616, 70.3306) centre (0, 0) ccw
  spline S214 degree 5 poles (42.1616, 70.3306) (42.1446, 70.3185) (42.1106, 70.2941) (42.0596, 70.2576) (41.9918, 70.2087) (41.9073, 70.1473) (41.823, 70.0857) (41.7391, 70.0239) (41.6553, 69.9619) (41.5719, 69.8996) (41.4887, 69.8371) (41.4058, 69.7743) (41.3232, 69.7114) (41.2408, 69.6481) (41.1587, 69.5847) (41.0769, 69.521) (40.9954, 69.457) (40.9142, 69.3929) (40.8333, 69.3285) (40.7526, 69.2638) (40.6723, 69.1989) (40.5922, 69.1337) (40.5125, 69.0683) (40.433, 69.0027) (40.3539, 68.9368) (40.2751, 68.8706) (40.1966, 68.8042) (40.1184, 68.7376) (40.0405, 68.6706) (39.963, 68.6035) (39.8857, 68.536) (39.8088, 68.4683) (39.7323, 68.4004) (39.6561, 68.3321) (39.5802, 68.2636) (39.5047, 68.1949) (39.4296, 68.1258) (39.3548, 68.0565) (39.2915, 67.9974) (39.2433, 67.9519) (39.21, 67.9204) (39.1915, 67.9029) (39.1878, 67.8994) knots -1 -1 -1 -1 -1 -1 -0.985714 -0.971429 -0.957143 -0.942857 -0.928571 -0.914286 -0.9 -0.885714 -0.871429 -0.857143 -0.842857 -0.828571 -0.814286 -0.8 -0.785714 -0.771429 -0.757143 -0.742857 -0.728571 -0.714286 -0.7 -0.685714 -0.671429 -0.657143 -0.642857 -0.628571 -0.614286 -0.6 -0.585714 -0.571429 -0.557143 -0.542857 -0.528571 -0.514286 -0.5 -0.485714 -0.471429 -0.467834 -0.467834 -0.467834 -0.467834 -0.467834 -0.467834
  spline S215 degree 3 poles (38.0098, 67.7523) (38.1234, 67.6886) (38.2483, 67.6476) (38.5068, 67.616) (38.6379, 67.6256) (38.8427, 67.6817) (38.9189, 67.7131) (39.0619, 67.7938) (39.1282, 67.8428) (39.1878, 67.8994) knots 0 0 0 0 0.039064 0.039064 0.078129 0.078129 0.102767 0.102767 0.127404 0.127404 0.127404 0.127404
  arc A108 (38.0098, 67.7523) -> (37.9083, 67.8091) centre (0, 0) ccw
  spline S216 degree 3 poles (37.4182, 68.8904) (37.391, 68.763) (37.389, 68.6316) (37.4355, 68.3754) (37.4836, 68.253) (37.598, 68.0741) (37.6506, 68.0106) (37.7701, 67.898) (37.8366, 67.8492) (37.9083, 67.8091) knots 0 0 0 0 0.039064 0.039064 0.078129 0.078129 0.102767 0.102767 0.127404 0.127404 0.127404 0.127404
  spline S217 degree 5 poles (37.4182, 68.8904) (37.4192, 68.8954) (37.4245, 68.9203) (37.434, 68.9652) (37.4475, 69.03) (37.4649, 69.1149) (37.4849, 69.2149) (37.5045, 69.315) (37.5237, 69.4153) (37.5425, 69.5158) (37.5608, 69.6164) (37.5788, 69.7172) (37.5963, 69.8182) (37.6135, 69.9192) (37.6302, 70.0204) (37.6466, 70.1218) (37.6626, 70.2233) (37.6782, 70.3249) (37.6934, 70.4267) (37.7082, 70.5286) (37.7227, 70.6307) (37.7368, 70.7328) (37.7505, 70.8351) (37.7639, 70.9376) (37.7769, 71.0401) (37.7895, 71.1428) (37.8018, 71.2456) (37.8137, 71.3485) (37.8253, 71.4515) (37.8365, 71.5546) (37.8474, 71.6579) (37.8579, 71.7612) (37.8681, 71.8647) (37.878, 71.9683) (37.8875, 72.072) (37.8966, 72.1758) (37.9054, 72.2797) (37.9139, 72.3837) (37.9221, 72.4878) (37.9283, 72.5712) (37.9329, 72.6338) (37.9358, 72.6755) (37.9373, 72.6964) knots 0.467834 0.467834 0.467834 0.467834 0.467834 0.467834 0.471429 0.485714 0.5 0.514286 0.528571 0.542857 0.557143 0.571429 0.585714 0.6 0.614286 0.628571 0.642857 0.657143 0.671429 0.685714 0.7 0.714286 0.728571 0.742857 0.757143 0.771429 0.785714 0.8 0.814286 0.828571 0.842857 0.857143 0.871429 0.885714 0.9 0.914286 0.928571 0.942857 0.957143 0.971429 0.985714 1 1 1 1 1 1
  arc A109 (37.9373, 72.6964) -> (36.5136, 73.4218) centre (0, 0) ccw
  spline S218 degree 5 poles (36.5136, 73.4218) (36.4976, 73.4083) (36.4656, 73.3814) (36.4176, 73.3409) (36.3538, 73.2869) (36.2744, 73.2191) (36.1952, 73.1511) (36.1164, 73.0829) (36.0378, 73.0144) (35.9595, 72.9458) (35.8815, 72.877) (35.8037, 72.8079) (35.7263, 72.7386) (35.6491, 72.6692) (35.5723, 72.5995) (35.4958, 72.5295) (35.4195, 72.4594) (35.3436, 72.389) (35.2679, 72.3185) (35.1926, 72.2477) (35.1176, 72.1767) (35.0429, 72.1054) (34.9686, 72.034) (34.8945, 71.9623) (34.8208, 71.8904) (34.7474, 71.8183) (34.6743, 71.7459) (34.6016, 71.6733) (34.5292, 71.6005) (34.4572, 71.5274) (34.3855, 71.4541) (34.3142, 71.3806) (34.2432, 71.3069) (34.1726, 71.2329) (34.1023, 71.1586) (34.0324, 71.0842) (33.9629, 71.0094) (33.8938, 70.9345) (33.8353, 70.8705) (33.7908, 70.8215) (33.7601, 70.7874) (33.7431, 70.7685) (33.7396, 70.7647) knots -1 -1 -1 -1 -1 -1 -0.985714 -0.971429 -0.957143 -0.942857 -0.928571 -0.914286 -0.9 -0.885714 -0.871429 -0.857143 -0.842857 -0.828571 -0.814286 -0.8 -0.785714 -0.771429 -0.757143 -0.742857 -0.728571 -0.714286 -0.7 -0.685714 -0.671429 -0.657143 -0.642857 -0.628571 -0.614286 -0.6 -0.585714 -0.571429 -0.557143 -0.542857 -0.528571 -0.514286 -0.5 -0.485714 -0.471429 -0.467834 -0.467834 -0.467834 -0.467834 -0.467834 -0.467834
  spline S219 degree 3 poles (32.5768, 70.5256) (32.695, 70.471) (32.8228, 70.44) (33.083, 70.4288) (33.2129, 70.4486) (33.4127, 70.5206) (33.4862, 70.5579) (33.6225, 70.6496) (33.6847, 70.7036) (33.7396, 70.7647) knots 0 0 0 0 0.039064 0.039064 0.078129 0.078129 0.102767 0.102767 0.127404 0.127404 0.127404 0.127404
  arc A110 (32.5768, 70.5256) -> (32.4711, 70.5744) centre (0, 0) ccw
  spline S220 degree 3 poles (31.8977, 71.6138) (31.8807, 71.4847) (31.889, 71.3535) (31.9555, 71.1017) (32.013, 70.9835) (32.141, 70.8142) (32.1984, 70.755) (32.3264, 70.6521) (32.3965, 70.6087) (32.4711, 70.5744) knots 0 0 0 0 0.039064 0.039064 0.078129 0.078129 0.102767 0.102767 0.127404 0.127404 0.127404 0.127404
  spline S221 degree 5 poles (31.8977, 71.6138) (31.8984, 71.6189) (31.9018, 71.6442) (31.9077, 71.6896) (31.9161, 71.7553) (31.9267, 71.8413) (31.9389, 71.9425) (31.9505, 72.0439) (31.9618, 72.1454) (31.9726, 72.2471) (31.983, 72.3488) (31.993, 72.4507) (32.0026, 72.5527) (32.0117, 72.6548) (32.0205, 72.757) (32.0289, 72.8594) (32.0368, 72.9618) (32.0444, 73.0644) (32.0516, 73.167) (32.0584, 73.2698) (32.0648, 73.3726) (32.0708, 73.4756) (32.0765, 73.5786) (32.0818, 73.6818) (32.0867, 73.785) (32.0912, 73.8884) (32.0954, 73.9918) (32.0992, 74.0953) (32.1027, 74.199) (32.1058, 74.3027) (32.1085, 74.4065) (32.1109, 74.5103) (32.1129, 74.6143) (32.1146, 74.7183) (32.116, 74.8224) (32.1169, 74.9266) (32.1176, 75.0309) (32.1179, 75.1353) (32.1178, 75.2397) (32.1175, 75.3233) (32.1172, 75.386) (32.1168, 75.4279) (32.1167, 75.4488) knots 0.467834 0.467834 0.467834 0.467834 0.467834 0.467834 0.471429 0.485714 0.5 0.514286 0.528571 0.542857 0.557143 0.571429 0.585714 0.6 0.614286 0.628571 0.642857 0.657143 0.671429 0.685714 0.7 0.714286 0.728571 0.742857 0.757143 0.771429 0.785714 0.8 0.814286 0.828571 0.842857 0.857143 0.871429 0.885714 0.9 0.914286 0.928571 0.942857 0.957143 0.971429 0.985714 1 1 1 1 1 1
  arc A111 (32.1167, 75.4488) -> (30.6404, 76.0603) centre (0, 0) ccw
  spline S222 degree 5 poles (30.6404, 76.0603) (30.6255, 76.0456) (30.5957, 76.0162) (30.5511, 75.9721) (30.4917, 75.9132) (30.4179, 75.8394) (30.3443, 75.7654) (30.271, 75.6912) (30.198, 75.6169) (30.1254, 75.5423) (30.053, 75.4675) (29.9809, 75.3926) (29.9091, 75.3175) (29.8377, 75.2421) (29.7666, 75.1666) (29.6957, 75.0909) (29.6252, 75.015) (29.555, 74.9389) (29.4852, 74.8626) (29.4156, 74.7861) (29.3464, 74.7095) (29.2776, 74.6326) (29.209, 74.5555) (29.1408, 74.4783) (29.073, 74.4008) (29.0055, 74.3231) (28.9383, 74.2452) (28.8715, 74.1672) (28.8051, 74.0889) (28.739, 74.0104) (28.6733, 73.9317) (28.6079, 73.8528) (28.543, 73.7737) (28.4784, 73.6944) (28.4141, 73.6149) (28.3503, 73.5352) (28.2869, 73.4552) (28.2238, 73.3751) (28.1706, 73.3067) (28.1301, 73.2543) (28.1021, 73.218) (28.0866, 73.1978) (28.0835, 73.1937) knots -1 -1 -1 -1 -1 -1 -0.985714 -0.971429 -0.957143 -0.942857 -0.928571 -0.914286 -0.9 -0.885714 -0.871429 -0.857143 -0.842857 -0.828571 -0.814286 -0.8 -0.785714 -0.771429 -0.757143 -0.742857 -0.728571 -0.714286 -0.7 -0.685714 -0.671429 -0.657143 -0.642857 -0.628571 -0.614286 -0.6 -0.585714 -0.571429 -0.557143 -0.542857 -0.528571 -0.514286 -0.5 -0.485714 -0.471429 -0.467834 -0.467834 -0.467834 -0.467834 -0.467834 -0.467834
  spline S223 degree 3 poles (26.943, 72.8642) (27.0652, 72.819) (27.195, 72.7981) (27.4552, 72.8073) (27.5832, 72.8373) (27.7767, 72.9248) (27.8471, 72.9677) (27.9757, 73.0698) (28.0335, 73.1286) (28.0835, 73.1937) knots 0 0 0 0 0.039064 0.039064 0.078129 0.078129 0.102767 0.102767 0.127404 0.127404 0.127404 0.127404
  arc A112 (26.943, 72.8642) -> (26.8339, 72.9045) centre (0, 0) ccw
  spline S224 degree 3 poles (26.1807, 73.8957) (26.1738, 73.7657) (26.1924, 73.6356) (26.2784, 73.3897) (26.345, 73.2764) (26.4859, 73.1176) (26.5478, 73.0631) (26.6835, 72.9706) (26.7568, 72.9328) (26.8339, 72.9045) knots 0 0 0 0 0.039064 0.039064 0.078129 0.078129 0.102767 0.102767 0.127404 0.127404 0.127404 0.127404
  spline S225 degree 5 poles (26.1807, 73.8957) (26.1809, 73.9008) (26.1823, 73.9263) (26.1846, 73.9721) (26.1878, 74.0382) (26.1917, 74.1248) (26.1959, 74.2267) (26.1995, 74.3286) (26.2028, 74.4307) (26.2056, 74.5329) (26.208, 74.6352) (26.2099, 74.7375) (26.2115, 74.8399) (26.2126, 74.9424) (26.2133, 75.045) (26.2136, 75.1477) (26.2136, 75.2505) (26.2131, 75.3533) (26.2122, 75.4562) (26.2109, 75.5592) (26.2092, 75.6622) (26.2072, 75.7653) (26.2047, 75.8685) (26.2019, 75.9718) (26.1987, 76.0751) (26.1951, 76.1785) (26.1912, 76.2819) (26.1868, 76.3854) (26.1821, 76.489) (26.1771, 76.5926) (26.1717, 76.6963) (26.1659, 76.8) (26.1598, 76.9038) (26.1533, 77.0077) (26.1464, 77.1116) (26.1393, 77.2155) (26.1317, 77.3195) (26.1238, 77.4236) (26.1156, 77.5277) (26.1087, 77.611) (26.1034, 77.6735) (26.0998, 77.7152) (26.098, 77.736) knots 0.467834 0.467834 0.467834 0.467834 0.467834 0.467834 0.471429 0.485714 0.5 0.514286 0.528571 0.542857 0.557143 0.571429 0.585714 0.6 0.614286 0.628571 0.642857 0.657143 0.671429 0.685714 0.7 0.714286 0.728571 0.742857 0.757143 0.771429 0.785714 0.8 0.814286 0.828571 0.842857 0.857143 0.871429 0.885714 0.9 0.914286 0.928571 0.942857 0.957143 0.971429 0.985714 1 1 1 1 1 1
  arc A113 (26.098, 77.736) -> (24.5784, 78.2298) centre (0, 0) ccw
  spline S226 degree 5 poles (24.5784, 78.2298) (24.5646, 78.214) (24.5372, 78.1824) (24.4962, 78.135) (24.4417, 78.0716) (24.3738, 77.9922) (24.3063, 77.9127) (24.239, 77.8329) (24.1721, 77.7531) (24.1055, 77.673) (24.0392, 77.5928) (23.9733, 77.5125) (23.9076, 77.4319) (23.8423, 77.3512) (23.7773, 77.2704) (23.7126, 77.1893) (23.6483, 77.1081) (23.5843, 77.0268) (23.5206, 76.9452) (23.4573, 76.8635) (23.3943, 76.7817) (23.3317, 76.6996) (23.2694, 76.6174) (23.2075, 76.535) (23.1459, 76.4525) (23.0847, 76.3697) (23.0239, 76.2868) (22.9634, 76.2038) (22.9033, 76.1205) (22.8436, 76.0371) (22.7843, 75.9535) (22.7253, 75.8697) (22.6667, 75.7858) (22.6086, 75.7016) (22.5508, 75.6173) (22.4934, 75.5328) (22.4364, 75.4482) (22.3799, 75.3633) (22.3322, 75.291) (22.2959, 75.2356) (22.2709, 75.1972) (22.257, 75.1758) (22.2542, 75.1715) knots -1 -1 -1 -1 -1 -1 -0.985714 -0.971429 -0.957143 -0.942857 -0.928571 -0.914286 -0.9 -0.885714 -0.871429 -0.857143 -0.842857 -0.828571 -0.814286 -0.8 -0.785714 -0.771429 -0.757143 -0.742857 -0.728571 -0.714286 -0.7 -0.685714 -0.671429 -0.657143 -0.642857 -0.628571 -0.614286 -0.6 -0.585714 -0.571429 -0.557143 -0.542857 -0.528571 -0.514286 -0.5 -0.485714 -0.471429 -0.467834 -0.467834 -0.467834 -0.467834 -0.467834 -0.467834
  spline S227 degree 3 poles (21.1431, 74.7535) (21.2684, 74.718) (21.3994, 74.7074) (21.6582, 74.737) (21.7834, 74.7769) (21.9695, 74.8793) (22.0363, 74.9276) (22.1565, 75.0395) (22.2095, 75.1026) (22.2542, 75.1715) knots 0 0 0 0 0.039064 0.039064 0.078129 0.078129 0.102767 0.102767 0.127404 0.127404 0.127404 0.127404
  arc A114 (21.1431, 74.7535) -> (21.0311, 74.7851) centre (0, 0) ccw
  spline S228 degree 3 poles (20.3022, 75.722) (20.3055, 75.5919) (20.3342, 75.4636) (20.4393, 75.2253) (20.5146, 75.1175) (20.6675, 74.9703) (20.7335, 74.9208) (20.876, 74.8392) (20.9521, 74.8073) (21.0311, 74.7851) knots 0 0 0 0 0.039064 0.039064 0.078129 0.078129 0.102767 0.102767 0.127404 0.127404 0.127404 0.127404
  spline S229 degree 5 poles (20.3022, 75.722) (20.302, 75.7272) (20.3014, 75.7526) (20.3001, 75.7985) (20.2981, 75.8646) (20.2952, 75.9512) (20.2913, 76.0531) (20.287, 76.1551) (20.2822, 76.2571) (20.277, 76.3592) (20.2714, 76.4613) (20.2653, 76.5635) (20.2588, 76.6658) (20.2519, 76.768) (20.2446, 76.8704) (20.2368, 76.9728) (20.2287, 77.0752) (20.2201, 77.1777) (20.2111, 77.2802) (20.2018, 77.3827) (20.192, 77.4853) (20.1819, 77.588) (20.1714, 77.6906) (20.1604, 77.7934) (20.1491, 77.8961) (20.1375, 77.9989) (20.1254, 78.1017) (20.113, 78.2045) (20.1002, 78.3074) (20.087, 78.4103) (20.0735, 78.5133) (20.0596, 78.6162) (20.0453, 78.7192) (20.0307, 78.8222) (20.0157, 78.9253) (20.0004, 79.0284) (19.9847, 79.1314) (19.9687, 79.2346) (19.9523, 79.3377) (19.939, 79.4202) (19.9288, 79.4821) (19.9219, 79.5234) (19.9185, 79.544) knots 0.467834 0.467834 0.467834 0.467834 0.467834 0.467834 0.471429 0.485714 0.5 0.514286 0.528571 0.542857 0.557143 0.571429 0.585714 0.6 0.614286 0.628571 0.642857 0.657143 0.671429 0.685714 0.7 0.714286 0.728571 0.742857 0.757143 0.771429 0.785714 0.8 0.814286 0.828571 0.842857 0.857143 0.871429 0.885714 0.9 0.914286 0.928571 0.942857 0.957143 0.971429 0.985714 1 1 1 1 1 1
  arc A115 (19.9185, 79.544) -> (18.3648, 79.9171) centre (0, 0) ccw
  spline S230 degree 5 poles (18.3648, 79.9171) (18.3523, 79.9002) (18.3275, 79.8666) (18.2903, 79.816) (18.2409, 79.7486) (18.1795, 79.6641) (18.1184, 79.5795) (18.0576, 79.4948) (17.9972, 79.4099) (17.9371, 79.3249) (17.8773, 79.2397) (17.8178, 79.1544) (17.7587, 79.069) (17.6999, 78.9834) (17.6414, 78.8977) (17.5833, 78.8119) (17.5256, 78.7259) (17.4681, 78.6397) (17.4111, 78.5534) (17.3544, 78.467) (17.298, 78.3805) (17.242, 78.2938) (17.1864, 78.2069) (17.1311, 78.1199) (17.0762, 78.0328) (17.0217, 77.9455) (16.9675, 77.8581) (16.9138, 77.7706) (16.8604, 77.6828) (16.8074, 77.595) (16.7548, 77.507) (16.7026, 77.4189) (16.6508, 77.3306) (16.5994, 77.2421) (16.5484, 77.1535) (16.4978, 77.0648) (16.4477, 76.9759) (16.398, 76.8869) (16.3561, 76.8111) (16.3242, 76.753) (16.3023, 76.7127) (16.2902, 76.6903) (16.2877, 76.6858) knots -1 -1 -1 -1 -1 -1 -0.985714 -0.971429 -0.957143 -0.942857 -0.928571 -0.914286 -0.9 -0.885714 -0.871429 -0.857143 -0.842857 -0.828571 -0.814286 -0.8 -0.785714 -0.771429 -0.757143 -0.742857 -0.728571 -0.714286 -0.7 -0.685714 -0.671429 -0.657143 -0.642857 -0.628571 -0.614286 -0.6 -0.585714 -0.571429 -0.557143 -0.542857 -0.528571 -0.514286 -0.5 -0.485714 -0.471429 -0.467834 -0.467834 -0.467834 -0.467834 -0.467834 -0.467834
  spline S231 degree 3 poles (15.2129, 76.1819) (15.3405, 76.1564) (15.472, 76.1561) (15.7276, 76.2059) (15.8494, 76.2555) (16.0268, 76.3722) (16.0896, 76.4256) (16.2007, 76.5465) (16.2486, 76.6136) (16.2877, 76.6858) knots 0 0 0 0 0.039064 0.039064 0.078129 0.078129 0.102767 0.102767 0.127404 0.127404 0.127404 0.127404
  arc A116 (15.2129, 76.1819) -> (15.0987, 76.2046) centre (0, 0) ccw
  spline S232 degree 3 poles (14.2985, 77.0815) (14.312, 76.952) (14.3508, 76.8264) (14.4742, 76.597) (14.5577, 76.4955) (14.7217, 76.3607) (14.7914, 76.3166) (14.9399, 76.2464) (15.0182, 76.2206) (15.0987, 76.2046) knots 0 0 0 0 0.039064 0.039064 0.078129 0.078129 0.102767 0.102767 0.127404 0.127404 0.127404 0.127404
  spline S233 degree 5 poles (14.2985, 77.0815) (14.298, 77.0866) (14.2953, 77.1119) (14.2905, 77.1575) (14.2833, 77.2234) (14.2736, 77.3095) (14.2617, 77.4107) (14.2494, 77.512) (14.2367, 77.6134) (14.2234, 77.7147) (14.2098, 77.8161) (14.1957, 77.9175) (14.1812, 78.0189) (14.1663, 78.1203) (14.151, 78.2218) (14.1352, 78.3232) (14.1191, 78.4247) (14.1025, 78.5262) (14.0855, 78.6277) (14.0681, 78.7292) (14.0504, 78.8307) (14.0322, 78.9322) (14.0136, 79.0338) (13.9947, 79.1353) (13.9754, 79.2369) (13.9557, 79.3384) (13.9356, 79.44) (13.9151, 79.5415) (13.8943, 79.6431) (13.8731, 79.7446) (13.8515, 79.8462) (13.8296, 79.9477) (13.8073, 80.0493) (13.7846, 80.1509) (13.7616, 80.2524) (13.7383, 80.354) (13.7146, 80.4555) (13.6905, 80.557) (13.6661, 80.6586) (13.6463, 80.7398) (13.6312, 80.8007) (13.6212, 80.8413) (13.6161, 80.8616) knots 0.467834 0.467834 0.467834 0.467834 0.467834 0.467834 0.471429 0.485714 0.5 0.514286 0.528571 0.542857 0.557143 0.571429 0.585714 0.6 0.614286 0.628571 0.642857 0.657143 0.671429 0.685714 0.7 0.714286 0.728571 0.742857 0.757143 0.771429 0.785714 0.8 0.814286 0.828571 0.842857 0.857143 0.871429 0.885714 0.9 0.914286 0.928571 0.942857 0.957143 0.971429 0.985714 1 1 1 1 1 1
  arc A117 (13.6161, 80.8616) -> (12.0379, 81.1116) centre (0, 0) ccw